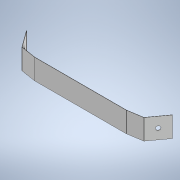
# Autodesk Inventor part: SIDE
Saved by Autodesk Inventor 2020 (Build 240168000, 168)
## iProperties
Created: 2022-07-14
Part Number: SIDE
Material: Generic
Document SubType Name: Sheet Metal
Designer: karimi2
Density: 1 g/cm^3
Sheet Metal Rule: Default_mm
Appearance: Default
Author: karimi2
Autodesk Inventor part; units mm, degrees
ref_plane "YZ Plane" through (0, 0, 0) normal (1, 0, 0) x (0, 1, 0)
ref_plane "XZ Plane" through (0, 0, 0) normal (0, 1, 0) x (-1, 0, 0)
ref_plane "XY Plane" through (0, 0, 0) normal (0, 0, 1) x (1, 0, 0)
sketch "Sketch1" plane through (0, 0, 0) normal (0, 0, 1) x (1, 0, 0)
  line L0 (0, 0) -> (-160, 0)
  line L1 (-160, 0) -> (-160, 40)
  line L2 (-160, 40) -> (0, 40)
  line L3 (0, 40) -> (0, 0) construction
  line L4 (0, 0) -> (160, 0)
  line L5 (160, 0) -> (160, 40)
  line L6 (160, 40) -> (0, 40)
  line L7 (-120, 40) -> (-120, 0)
  line L8 (120, 40) -> (120, 0)
  line L9 (90, 40) -> (90, 0)
  line L10 (-90, 40) -> (-90, 0)
  circle A0 centre (140, 20) radius 4
  circle A1 centre (-140, 20) radius 4
  dimension "d0" = 160
  dimension "d1" = 40
  dimension "d2" = 40
  dimension "d3" = 40
  dimension "d4" = 30
  dimension "d5" = 30
  dimension "d43" = 20
  dimension "d44" = 8
  dimension "d45" = 20
  dimension "d46" = 20
  constraints: 22 end point, 8 point on line, 4 perpendicular, 3 parallel, 2 centre point, 2 symmetric about line, 1 equal radius, 1 horizontal, 1 horizontal alignment
  measures "d0" distance of L1.end L2.end
  measures "d1" distance of L0.end L1.end
  measures "d2" distance from line of L0.end L7
  measures "d3" distance between parallel lines of L5 L8
  measures "d4" distance between parallel lines of L10 L7
  measures "d5" distance between parallel lines of L8 L9
  measures "d43" distance from line of L4 A0.centre
  measures "d44" diameter of A0
  measures "d45" distance from line of L1 A1.centre
  measures "d46" distance from line of L8 A0.centre
extrude "Plate3" add sketch "Sketch1" along normal blind 0.5
fold "Fold9" angle 45 bend radius 0.5 thickness 0.5 k factor 0.44 line from (-120, 40, 0) to (-120, 0, 0) line at bend centre moving side (-1, 0, 0) folds toward (0, 0, -1)
fold "Fold10" angle 9 bend radius 0.5 thickness 0.5 k factor 0.44 line from (-90, 40, 0) to (-90, 0, 0) line at bend centre moving side (-1, 0, 0) folds toward (0, 0, -1)
fold "Fold11" angle 45 bend radius 0.5 thickness 0.5 k factor 0.44 line from (120, 40, 0) to (120, 0, 0) line at bend centre moving side (1, 0, 0) folds toward (0, 0, -1)
fold "Fold12" angle 9 bend radius 0.5 thickness 0.5 k factor 0.44 line from (90, 40, 0) to (90, 0, 0) line at bend centre moving side (1, 0, 0) folds toward (0, 0, -1)
equation "\"d72\" = Thickness"
equation "\"d73\" = BendReliefWidth"
equation "\"d74\" = BendReliefDepth"
equation "\"d75\" = MinimumRemnant"
equation "\"d76\" = TransitionRadius"
equation "\"d78\" = BendRadius"
equation "\"d79\" = BendReliefWidth"
equation "\"d80\" = BendReliefDepth"
equation "\"d81\" = MinimumRemnant"
equation "\"d82\" = TransitionRadius"
equation "\"d84\" = BendRadius"
equation "\"d85\" = BendReliefWidth"
equation "\"d86\" = BendReliefDepth"
equation "\"d87\" = MinimumRemnant"
equation "\"d88\" = TransitionRadius"
equation "\"d90\" = BendRadius"
equation "\"d91\" = BendReliefWidth"
equation "\"d92\" = BendReliefDepth"
equation "\"d93\" = MinimumRemnant"
equation "\"d94\" = TransitionRadius"
equation "\"d96\" = BendRadius"
equation "\"BendRadius\" = Thickness"
equation "\"BendReliefWidth\" = Thickness"
equation "\"BendReliefDepth\" = 0.5 * Thickness"
equation "\"CornerReliefSize\" = 4 * Thickness"
equation "\"MinimumRemnant\" = 2 * Thickness"
equation "\"TransitionRadius\" = BendRadius"
equation "\"JacobiRadiusSize\" = BendRadius"
equation "\"GapSize\" = Thickness"
equation "\"Thickness\" = 0.5"
body "Solid3"
